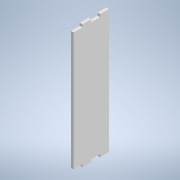
# Autodesk Inventor part: voorruit
Saved by Autodesk Inventor 2021 (Build 250183000, 183)
## iProperties
Created: 2022-02-02
Part Number: voorruit
Material: Generic
Document SubType Name: Modeling
Designer: ryan
Density: 1 g/cm^3
Appearance: Default
Author: ryan
Autodesk Inventor part; units mm, degrees
ref_plane "YZ Plane" through (0, 0, 0) normal (1, 0, 0) x (0, 1, 0)
ref_plane "XZ Plane" through (0, 0, 0) normal (0, 1, 0) x (-1, 0, 0)
ref_plane "XY Plane" through (0, 0, 0) normal (0, 0, 1) x (1, 0, 0)
sketch "Sketch1" plane through (0, 0, 0) normal (1, 0, 0) x (0, 1, 0)
  line L0 (0, 0) -> (0, 10)
  line L1 (0, 10) -> (0, 20)
  line L2 (0, 20) -> (0, 30)
  line L3 (0, 30) -> (0, 40)
  line L4 (0, 40) -> (-70, 40)
  line L5 (-70, 40) -> (-70, 0)
  line L6 (-70, 0) -> (0, 0)
  line L7 (0, 0) -> (0, 40)
  line L8 (0, 40) -> (-3, 40)
  line L9 (-3, 40) -> (-3, 30)
  line L10 (-3, 30) -> (-3, 20)
  line L11 (-3, 20) -> (-3, 10)
  line L12 (-3, 10) -> (-3, 0)
  line L13 (-3, 30) -> (0, 30)
  line L14 (-3, 20) -> (0, 20)
  line L15 (-3, 10) -> (0, 10)
  dimension "d0" = 10
  dimension "d1" = 10
  dimension "d2" = 10
  dimension "d3" = 10
  dimension "d4" = 70
  dimension "d5" = 40
  dimension "d6" = 3
  dimension "d7" = 10
  dimension "d8" = 10
  dimension "d9" = 10
  dimension "d10" = 10
  constraints: 32 end point, 7 point on line, 2 parallel, 2 perpendicular, 1 horizontal, 1 vertical
  measures "d0" distance of L0.start L0.end
  measures "d1" distance of L0.end L1.end
  measures "d2" distance of L1.end L2.end
  measures "d3" distance of L2.end L3.end
  measures "d4" distance of L6.end L5.end
  measures "d5" distance of L5.end L4.end
  measures "d6" distance of L3.end L8.end
  measures "d7" distance of L8.end L9.end
  measures "d8" distance of L9.end L10.end
  measures "d9" distance of L10.end L11.end
  measures "d10" distance of L11.end L12.end
extrude "Extrusion1" add sketch "Sketch1" against normal blind 3 contours L6 L12 L15 L0 | L6 L5 L4 L9 L10 L11 L12 | L14 L10 L13 L2
mirror "Mirror1" about plane through (0, -70, 0) normal (0, -1, 0) of "Extrusion1"
body "Solid1"
